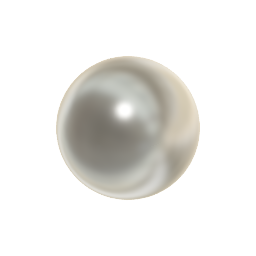
Bearing Assembly_ (Autodesk Fusion 360 archive; units mm, degrees)
design "Bearing Assembly Ball"
Autodesk Fusion 360 part; units mm, degrees
sketch "Sketch1" plane through (0, 0, 0) normal (0, 1, 0) x (1, 0, 0)
  arc A0 (0, -3) -> (0, 3) centre (0, 0) ccw
  line L0 (0, -3) -> (0, 3)
  dimension "d1" = 3
  constraint coincident A0.centre origin
  constraint vertical L0
  measures "d1" radius of A0
revolve "Revolve1" add sketch "Sketch1" angle 360 about axis through (0, 0, 3) along (0, 0, -1)

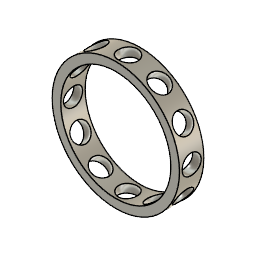
design "Bearing Assembly Cage"
Autodesk Fusion 360 part; units mm, degrees
sketch "Sketch1" plane through (0, 0, 0) normal (0, 1, 0) x (1, 0, 0)
  circle A0 centre (0, 0) radius 18.25
  circle A1 centre (0, 0) radius 15.75
  dimension "d1" = 36.5
  dimension "d2" = 31.5
  constraint coincident A0.centre A1.centre
  constraint concentric A0 A1
  measures "d1" diameter of A0
  measures "d2" diameter of A1
extrude "Extrude1" add sketch "Sketch1" along normal mid plane 7
sketch "Sketch3" plane through (0, 0, 0) normal (0, 1, 0) x (1, 0, 0)
  line L0 (0, 0) -> (0, -29.5716) construction
  arc A0 (0, -14) -> (0, -20) centre (0, -17) ccw
  line L1 (0, -20) -> (0, -14)
  dimension "d5" = 3
  dimension "d6" = 17
  constraint coincident L0.start origin
  constraint vertical L0
  constraint coincident L0 A0.start
  constraint coincident L0 A0.end
  constraint coincident L0 A0.centre
  measures "d5" radius of A0
  measures "d6" distance of L0.start A0.centre
revolve "Revolve1" cut sketch "Sketch3" angle 360 about axis through (0, 0, 0) along (0, 0, 1)
pattern_circular "C-Pattern1" count 12 over 360 about axis through (0, -3.5, 0) along (0, 1, 0) of "Revolve1"

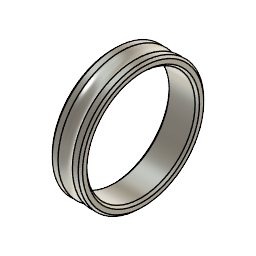
design "Bearing Assembly Inner Ring"
Autodesk Fusion 360 part; units mm, degrees
sketch "Sketch2" plane through (0, 0, 0) normal (0, 1, 0) x (1, 0, 0)
  line L0 (0, 0) -> (0, -17.2519) construction
  line L1 (0, -17.2519) -> (0, 0) construction
  line L2 (0, 0) -> (-10.0877, 0) construction
  line L3 (-1.6583, -14.5) -> (-3.5, -14.5)
  line L4 (-3.5, -14.5) -> (-3.5, -12.5)
  line L5 (-3.5, -12.5) -> (3.5, -12.5)
  line L6 (3.5, -12.5) -> (3.5, -14.5)
  line L7 (3.5, -14.5) -> (1.6583, -14.5)
  arc A0 (1.6583, -14.5) -> (-1.6583, -14.5) centre (0, -17) ccw
  dimension "d7" = 29
  dimension "d8" = 25
  dimension "d9" = 7
  dimension "d10" = 3
  dimension "d12" = 17
  constraint coincident L0.start L1.end
  constraint vertical L0
  constraint perpendicular L1 L2
  constraint perpendicular L3 L4
  constraint perpendicular L4 L5
  constraint perpendicular L5 L6
  constraint perpendicular L4 L7
  constraint symmetric L0 L3 L7
  constraint equal L3 L7
  measures "d9" distance of L4 L6
  measures "d10" radius of A0
  measures "d12" vertical distance of L0.start A0.centre
revolve "Revolve1" add sketch "Sketch2" angle 360 about axis through (1.75, 0, 0) along (1, 0, 0)
chamfer "Chamfer1" distance 0.5 angle 45 4 edges at (-3.5, -5.2434, -13.5187) (3.5, -5.2434, -13.5187) (-3.5, -4.5202, -11.6541) (3.5, -4.5202, -11.6541)

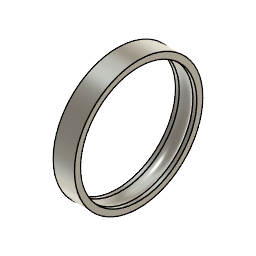
design "Bearing Assembly Outer Ring"
Autodesk Fusion 360 part; units mm, degrees
sketch "Sketch1" plane through (0, 0, 0) normal (0, 1, 0) x (1, 0, 0)
  line L0 (0, 0) -> (-46.3404, 0) construction
  line L1 (-46.3404, 0) -> (0, 0) construction
  line L2 (0, 0) -> (0, -63.877) construction
  line L3 (-2.2361, -19) -> (-3.5, -19)
  line L4 (-3.5, -19) -> (-3.5, -21)
  line L5 (-3.5, -21) -> (3.5, -21)
  line L6 (3.5, -21) -> (3.5, -19)
  line L7 (3.5, -19) -> (2.2361, -19)
  arc A0 (-2.2361, -19) -> (2.2361, -19) centre (0, -17) ccw
  dimension "d1" = 3
  dimension "d2" = 7
  dimension "d3" = 42
  dimension "d4" = 38
  dimension "d5" = 17
  constraint coincident L0.start L1.end
  constraint horizontal L0
  constraint perpendicular L0 L2
  constraint perpendicular L2 L3
  constraint perpendicular L3 L4
  constraint perpendicular L2 L5
  constraint perpendicular L5 L6
  constraint perpendicular L6 L7
  constraint equal L3 L7
  constraint horizontal L3.start L7.end
  measures "d1" radius of A0
  measures "d2" distance of L4.end L5.end
  measures "d5" distance of L0.start A0.centre
revolve "Revolve1" add sketch "Sketch1" angle 360 about axis through (1.75, 0, 0) along (1, 0, 0)
